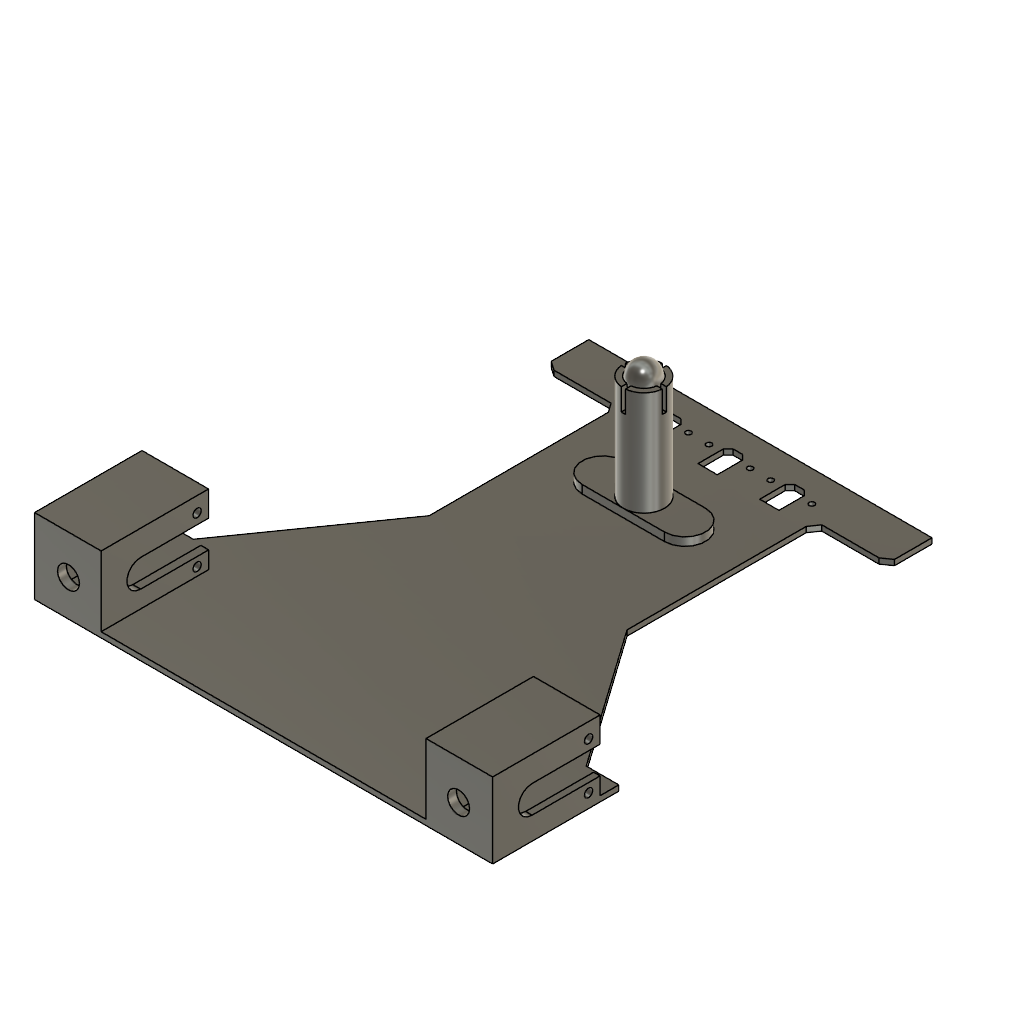
line follower (Autodesk Fusion 360 design; units mm, degrees)
part number: 2026-04-11-10-52-49-664
Autodesk Fusion 360 part; units mm, degrees
note: some values were not read from the file. Set by a fixed rule: which sketch regions a step uses.
sketch "Sketch1" plane through (0, 0, 0) normal (0, 0, 1) x (1, 0, 0)
  line L0 (0, 0) -> (83.525, 0)
  line L1 (83.525, 0) -> (83.525, 46.04)
  line L2 (83.525, 46.04) -> (71.635, 46.04)
  line L3 (71.635, 46.04) -> (36.0768, 96.4755)
  line L4 (36.0768, 96.4755) -> (36.0768, 161.7955)
  line L5 (36.0768, 161.7955) -> (38.4036, 165.1348)
  line L6 (38.4036, 165.1348) -> (59.2636, 165.1348)
  line L7 (59.2636, 165.1348) -> (62.59, 167.48)
  line L8 (62.59, 167.48) -> (62.59, 181.19)
  line L9 (62.59, 181.19) -> (0, 181.19)
  line L10 (0, 181.19) -> (0, 0)
  dimension "d3" = 62.59
  dimension "d4" = 181.19
  dimension "d5" = 13.71
  dimension "d8" = 65.32
  dimension "d9" = 46.04
  dimension "d10" = 83.525
  dimension "d11" = 11.89
  dimension "d12" = 61.71
  dimension "d15" = 4.07
  dimension "d16" = 20.86
  dimension "d18" = 4.07
  constraint coincident L0.start L10.end
  constraint horizontal L0
  constraint perpendicular L0 L1
  constraint perpendicular L1 L2
  constraint perpendicular L0 L4
  constraint perpendicular L4 L6
  constraint perpendicular L3 L7
  constraint perpendicular L0 L8
  constraint perpendicular L8 L9
  constraint perpendicular L0 L10
  measures "d3" distance of L8.end L9.end
  measures "d4" distance of L9.end L0.start
  measures "d5" distance of L7.end L8.end
  measures "d8" distance of L3.end L4.end
  measures "d9" distance of L0.end L1.end
  measures "d10" distance of L0.start L0.end
  measures "d11" distance of L1.end L2.end
  measures "d12" distance of L2.end L3.end
  measures "d15" distance of L6.end L7.end
  measures "d16" distance of L5.end L6.end
  measures "d18" distance of L4.end L5.end
extrude "Extrude1" add sketch "Sketch1" along normal blind 2 makes body 1
mirror "Mirror1" about plane through (0, 0, 0) normal (1, 0, 0) of bodies 1 merged
sketch "Sketch3" plane through (83.525, 0, 0) normal (1, 0, 0) x (0, 1, 0)
  line L0 (0, 0) -> (46.04, 0)
  line L1 (46.04, 0) -> (46.04, 2)
  line L2 (46.04, 2) -> (0, 2)
  line L3 (0, 2) -> (0, 0)
  line L4 (46.04, 2) -> (96.4755, 2)
  line L5 (19.51, 20.5) -> (19.51, 42)
  line L6 (26.51, 20.5) -> (26.51, 42)
  line L7 (19.51, 42) -> (26.51, 42)
  arc A0 (19.51, 20.5) -> (26.51, 20.5) centre (23.01, 20.5) ccw
  dimension "d28" = 7
  dimension "d29" = 18.5
  constraint tangent L5 A0
  constraint tangent L6 A0
  measures "d28" diameter of A0
  measures "d29" distance of A0.centre L4
extrude "Extrude3" cut sketch "Sketch3" against normal blind 2 contours L5 L6 L7 A0 bodies 1
mirror "Mirror2" [no effect]
sketch "Sketch4" plane through (0, 0, 2) normal (0, 0, 1) x (-1, 0, 0)
  line L0 (83.525, -46.04) -> (83.525, 0)
  line L1 (83.525, 0) -> (-83.525, 0)
  line L2 (-83.525, 0) -> (-83.525, -46.04)
  line L3 (-83.525, -46.04) -> (-71.635, -46.04)
  line L4 (-71.635, -46.04) -> (-36.0768, -96.4755)
  line L5 (-36.0768, -96.4755) -> (-36.0768, -161.7955)
  line L6 (-36.0768, -161.7955) -> (-38.4036, -165.1348)
  line L7 (-38.4036, -165.1348) -> (-59.2636, -165.1348)
  line L8 (-59.2636, -165.1348) -> (-62.59, -167.48)
  line L9 (-62.59, -167.48) -> (-62.59, -181.19)
  line L10 (-62.59, -181.19) -> (62.59, -181.19)
  line L11 (62.59, -181.19) -> (62.59, -167.48)
  line L12 (62.59, -167.48) -> (59.2636, -165.1348)
  line L13 (59.2636, -165.1348) -> (38.4036, -165.1348)
  line L14 (38.4036, -165.1348) -> (36.0768, -161.7955)
  line L15 (36.0768, -161.7955) -> (36.0768, -96.4755)
  line L16 (36.0768, -96.4755) -> (71.635, -46.04)
  line L17 (71.635, -46.04) -> (83.525, -46.04)
  line L18 (-3.5, -161.94) -> (3.5, -161.94)
  line L19 (3.5, -161.94) -> (3.5, -172.94)
  line L20 (3.5, -172.94) -> (-3.5, -172.94)
  line L21 (-3.5, -172.94) -> (-3.5, -161.94)
  line L22 (-3.5, -161.94) -> (3.5, -172.94) construction
  line L23 (3.5, -161.94) -> (-3.5, -172.94) construction
  line L24 (-3.5, -171.19) -> (-1.75, -172.94)
  circle A0 centre (-7.5, -169.94) radius 1
  line L25 (0, -167.44) -> (0, -181.19) construction
  circle A1 centre (7.5, -169.94) radius 1
  line L26 (3.5, -171.19) -> (1.75, -172.94)
  circle A2 centre (-30, -169.94) radius 1
  circle A3 centre (-15, -169.94) radius 1
  line L27 (-19, -161.94) -> (-19, -172.94)
  line L28 (-19, -172.94) -> (-26, -172.94)
  line L29 (-26, -172.94) -> (-26, -161.94)
  line L30 (-26, -171.19) -> (-24.25, -172.94)
  line L31 (-26, -161.94) -> (-19, -172.94) construction
  line L32 (-19, -171.19) -> (-20.75, -172.94)
  line L33 (-26, -161.94) -> (-19, -161.94)
  line L34 (-19, -161.94) -> (-26, -172.94) construction
  circle A4 centre (15, -169.94) radius 1
  circle A5 centre (30, -169.94) radius 1
  line L35 (26, -161.94) -> (26, -172.94)
  line L36 (26, -172.94) -> (19, -172.94)
  line L37 (19, -172.94) -> (19, -161.94)
  line L38 (19, -171.19) -> (20.75, -172.94)
  line L39 (19, -161.94) -> (26, -172.94) construction
  line L40 (26, -171.19) -> (24.25, -172.94)
  line L41 (19, -161.94) -> (26, -161.94)
  line L42 (26, -161.94) -> (19, -172.94) construction
  point P0 (0, -167.44)
  point P1 (-22.5, -167.44)
  point P2 (-22.5, -167.44)
  point P3 (22.5, -167.44)
  point P4 (22.5, -167.44)
  dimension "d34" = 7
  dimension "d35" = 11
  dimension "d36" = 8.25
  dimension "d37" = 1.75
  dimension "d38" = 1.75
  dimension "d39" = 2
  dimension "d40" = 11.25
  dimension "d41" = 4
  dimension "d44" = 22.5
  dimension "d45" = 0
  constraint horizontal L18
  constraint perpendicular L18 L19
  constraint parallel L18 L20
  constraint parallel L19 L21
  constraint coincident L22 P0
  constraint coincident L23 P0
  constraint coincident L21 L24.start
  constraint coincident L20 L24.end
  constraint coincident P0 L25.start
  constraint midpoint L10 L25.end
  constraint perpendicular L10 L25
  constraint symmetric L24.start L25 L26.start
  constraint symmetric L24.end L25 L26.end
  constraint symmetric A0 L25 A1
  measures "d34" distance of L18.start L18.end
  measures "d35" distance of L18.end L19.end
  measures "d36" distance of L10 L20
  measures "d37" distance of L20.end L24.end
  measures "d38" distance of L20.end L24.start
  measures "d39" diameter of A0
  measures "d40" distance of L10 A0.centre
  measures "d41" distance of L21 A0.centre
extrude "Extrude4" cut sketch "Sketch4" against normal blind 2 contours L18 L19 L20 L21 L24 L26 | A0 | A1 | A2 | A3 | L27 L28 L29 L30 L32 L33 | A4 | A5 | L35 L36 L37 L38 L40 L41 bodies 1
sketch "Sketch5" plane through (83.525, 0, 0) normal (1, 0, 0) x (0, 1, 0)
  line L0 (0, 0) -> (46.04, 0)
  line L1 (46.04, 0) -> (46.04, 2)
  line L2 (46.04, 2) -> (0, 2)
  line L3 (0, 2) -> (0, 0)
  line L4 (0, 2) -> (24.3, 2)
  line L5 (24.3, 2) -> (24.3, 27.5)
  line L6 (24.3, 27.5) -> (0, 27.5)
  line L7 (0, 27.5) -> (0, 2)
  circle A0 centre (11.9, 13.25) radius 4
  dimension "d48" = 24.3
  dimension "d49" = 25.5
  dimension "d50" = 8
  dimension "d51" = 14.25
  dimension "d53" = 11.9
  constraint horizontal L4
  constraint vertical L5
  constraint horizontal L6
  constraint vertical L7
  constraint coincident L2.end L3.start
  measures "d48" distance of L5.end L6.end
  measures "d49" distance of L2.end L6.end
  measures "d50" diameter of A0
  measures "d51" distance of L6 A0.centre
  measures "d53" distance of L7 A0.centre
extrude "Extrude5" add sketch "Sketch5" against normal blind 39.2 separate body contours L2 L4 L5 L6 L7 makes body 2
sketch "Sketch6" plane through (0, 0, 0) normal (0, -1, 0) x (1, 0, 0)
  line L0 (83.525, 2) -> (83.525, 27.5)
  line L1 (83.525, 27.5) -> (44.325, 27.5)
  line L2 (44.325, 27.5) -> (44.325, 2)
  line L3 (44.325, 2) -> (83.525, 2)
  line L4 (44.325, 8.25) -> (69.125, 8.25)
  arc A0 (69.125, 8.25) -> (69.125, 18.25) centre (69.125, 13.25) ccw
  line L5 (69.125, 18.25) -> (44.325, 18.25)
  arc A1 (44.325, 18.25) -> (44.325, 8.25) centre (44.325, 13.25) ccw
  line L6 (44.325, 13.25) -> (69.125, 13.25) construction
  circle A2 centre (48.525, 22) radius 1.5
  circle A3 centre (48.525, 5) radius 1.5
  dimension "d56" = 6.25
  dimension "d57" = 5
  dimension "d58" = 24.8
  dimension "d59" = 3
  dimension "d60" = 3
  dimension "d61" = 4.2
  dimension "d62" = 4.2
  dimension "d63" = 3
  dimension "d64" = 3.75
  constraint tangent L4 A0
  constraint tangent A0 L5
  constraint parallel L4 L5
  constraint tangent L5 A1
  constraint tangent L4 A1
  constraint perpendicular L2 L6
  constraint coincident L2 A1.centre
  measures "d56" distance of L3 L4
  measures "d57" radius of A0
  measures "d58" distance of A1.centre A0.centre
  measures "d59" diameter of A2
  measures "d60" diameter of A3
  measures "d61" distance of L2 A3.centre
  measures "d62" distance of L2 A2.centre
  measures "d63" distance of L3 A3.centre
  measures "d64" distance of L5 A2.centre
extrude "Extrude6" cut sketch "Sketch6" against normal blind 25 contours L2 L4 A0 L5 | A2 | A3 bodies 2
move_body "Move1" bodies 2 to x (0, -1, 0) y (1, 0, 0) z (0, 0, 1) at (83.525, 83.525, 0)
move_body "Move2" bodies 2 to x (1, 0, 0) y (0, 1, 0) z (0, 0, 1) at (-25, 0, 0)
move_body "Move3" bodies 2 to x (1, 0, 0) y (0, 1, 0) z (0, 0, 1) at (0.7, 0, 0)
sketch "Sketch7" plane through (0, 39.2, 0) normal (0, 1, 0) x (-1, 0, 0)
  line L0 (-59.225, 8.25) -> (-83.525, 8.25)
  line L1 (-83.525, 8.25) -> (-83.525, 2)
  line L2 (-83.525, 2) -> (-59.225, 2)
  line L3 (-59.225, 2) -> (-59.225, 8.25)
  line L4 (-81.175, 2) -> (-62.075, 2)
  line L5 (-62.075, 2) -> (-62.075, 24.65)
  line L6 (-62.075, 24.65) -> (-81.175, 24.65)
  line L7 (-81.175, 24.65) -> (-81.175, 2)
  dimension "d71" = 2.85
  dimension "d72" = 2.35
  dimension "d73" = 22.65
  constraint horizontal L4
  constraint vertical L5
  constraint horizontal L6
  constraint vertical L7
  constraint coincident L2 L4.start
  measures "d71" distance of L3 L5
  measures "d72" distance of L1 L7
  measures "d73" distance of L4 L6
extrude "Extrude7" cut sketch "Sketch7" against normal blind 36 contours L0 L2 L4 L5 L7 | L0 L5 L6 L7 bodies 2
mirror "Mirror3" about plane through (0, 0, 0) normal (1, 0, 0) of bodies 2 makes body 3
sketch "Sketch8" plane through (0, 0, 2) normal (0, 0, 1) x (-1, 0, 0)
  circle A0 centre (15, -169.94) radius 1
  line L0 (1.75, -172.94) -> (-1.75, -172.94)
  line L1 (-1.75, -172.94) -> (-3.5, -171.19)
  line L2 (-3.5, -171.19) -> (-3.5, -161.94)
  line L3 (-3.5, -161.94) -> (3.5, -161.94)
  line L4 (3.5, -161.94) -> (3.5, -171.19)
  line L5 (3.5, -171.19) -> (1.75, -172.94)
  circle A1 centre (-30, -169.94) radius 1
  circle A2 centre (7.5, -169.94) radius 1
  line L6 (24.25, -172.94) -> (20.75, -172.94)
  line L7 (20.75, -172.94) -> (19, -171.19)
  line L8 (19, -171.19) -> (19, -161.94)
  line L9 (19, -161.94) -> (26, -161.94)
  line L10 (26, -161.94) -> (26, -171.19)
  line L11 (26, -171.19) -> (24.25, -172.94)
  circle A3 centre (-15, -169.94) radius 1
  line L12 (-20.75, -172.94) -> (-24.25, -172.94)
  line L13 (-24.25, -172.94) -> (-26, -171.19)
  line L14 (-26, -171.19) -> (-26, -161.94)
  line L15 (-26, -161.94) -> (-19, -161.94)
  line L16 (-19, -161.94) -> (-19, -171.19)
  line L17 (-19, -171.19) -> (-20.75, -172.94)
  circle A4 centre (-7.5, -169.94) radius 1
  circle A5 centre (30, -169.94) radius 1
  line L18 (83.525, 0) -> (-83.525, 0)
  line L19 (-83.525, 0) -> (-83.525, -46.04)
  line L20 (-83.525, -46.04) -> (-71.635, -46.04)
  line L21 (-71.635, -46.04) -> (-36.0768, -96.4755)
  line L22 (-36.0768, -96.4755) -> (-36.0768, -161.7955)
  line L23 (-36.0768, -161.7955) -> (-38.4036, -165.1348)
  line L24 (-38.4036, -165.1348) -> (-59.2636, -165.1348)
  line L25 (-59.2636, -165.1348) -> (-62.59, -167.48)
  line L26 (-62.59, -167.48) -> (-62.59, -181.19)
  line L27 (-62.59, -181.19) -> (62.59, -181.19)
  line L28 (62.59, -181.19) -> (62.59, -167.48)
  line L29 (62.59, -167.48) -> (59.2636, -165.1348)
  line L30 (59.2636, -165.1348) -> (38.4036, -165.1348)
  line L31 (38.4036, -165.1348) -> (36.0768, -161.7955)
  line L32 (36.0768, -161.7955) -> (36.0768, -96.4755)
  line L33 (36.0768, -96.4755) -> (71.635, -46.04)
  line L34 (71.635, -46.04) -> (83.525, -46.04)
  line L35 (83.525, -46.04) -> (83.525, 0)
  line L36 (15, -131.19) -> (-15, -131.19)
  arc A6 (-15, -131.19) -> (-15, -146.19) centre (-15, -138.69) ccw
  line L37 (-15, -146.19) -> (15, -146.19)
  arc A7 (15, -146.19) -> (15, -131.19) centre (15, -138.69) ccw
  line L38 (15, -138.69) -> (-15, -138.69) construction
  point P0 (0, -138.69)
  dimension "d78" = 15
  dimension "d79" = 35
  constraint tangent L36 A6
  constraint tangent A6 L37
  constraint parallel L36 L37
  constraint tangent L37 A7
  constraint tangent L36 A7
  constraint perpendicular L22 L38
  constraint midpoint L38 P0
  measures "d78" diameter of A6
  measures "d79" distance of L27 L37
extrude "Extrude8" add sketch "Sketch8" along normal blind 3 contours L36 A6 L37 A7 bodies 1
sketch "Sketch9" plane through (0, 0, 5) normal (0, 0, 1) x (-1, 0, 0)
  arc A0 (15, -146.19) -> (15, -131.19) centre (15, -138.69) ccw
  line L0 (15, -131.19) -> (-15, -131.19)
  arc A1 (-15, -131.19) -> (-15, -146.19) centre (-15, -138.69) ccw
  line L1 (-15, -146.19) -> (15, -146.19)
  circle A2 centre (0, -138.69) radius 7.5
  dimension "d82" = 15
  dimension "d83" = 7.5
  measures "d82" diameter of A2
  measures "d83" distance of L1 A2.centre
extrude "Extrude9" add sketch "Sketch9" along normal blind 38 separate body contours A2 makes body 4
sphere "SpherePrimitive1" cut diameter 11 placed x (-1, 0, 0) y (0, -1, 0) z (0, 0, 1) at (0, 138.69, 43) bodies 4
sketch "Sketch11" plane through (0, 0, 43) normal (0, 0, 1) x (-1, 0, 0)
  circle A0 centre (0, -138.69) radius 5.5
  circle A1 centre (0, -138.69) radius 7.5
  line L0 (-0.75, -146.19) -> (0.75, -146.19)
  line L1 (0.75, -146.19) -> (0.75, -131.19)
  line L2 (0.75, -131.19) -> (-0.75, -131.19)
  line L3 (-0.75, -131.19) -> (-0.75, -146.19)
  line L4 (-0.75, -146.19) -> (0.75, -131.19) construction
  line L5 (0.75, -146.19) -> (-0.75, -131.19) construction
  line L6 (-7.5, -137.94) -> (7.5, -137.94)
  line L7 (7.5, -137.94) -> (7.5, -139.44)
  line L8 (7.5, -139.44) -> (-7.5, -139.44)
  line L9 (-7.5, -139.44) -> (-7.5, -137.94)
  line L10 (-7.5, -137.94) -> (7.5, -139.44) construction
  line L11 (7.5, -137.94) -> (-7.5, -139.44) construction
  point P0 (0, -138.69)
  point P1 (0, -138.69)
  dimension "d87" = 15
  dimension "d88" = 15
  dimension "d89" = 1.5
  dimension "d90" = 1.5
  constraint horizontal L0
  constraint perpendicular L0 L1
  constraint parallel L0 L2
  constraint parallel L1 L3
  constraint coincident L4 P1
  constraint coincident L5 P1
  constraint coincident P0 A0.centre
  constraint horizontal L6
  constraint perpendicular L6 L7
  constraint parallel L6 L8
  constraint parallel L7 L9
  constraint coincident L10 P1
  constraint coincident L11 P1
  constraint coincident P1 P0
  measures "d87" distance of L0.end L1.end
  measures "d88" distance of L6.start L6.end
  measures "d89" distance of L0.start L0.end
  measures "d90" distance of L6.start L8.end
extrude "Extrude10" cut sketch "Sketch11" against normal blind 8 contours A0 L1 L6 L8 | A0 A1 L6 L8 | A0 L1 L3 L6 | A0 A1 L1 L3 | L1 L3 L6 L8 | A0 A1 L1 L3 | A0 L1 L3 L8 | A0 L3 L6 L8 | A0 A1 L6 L8 bodies 4
sphere "SpherePrimitive2" add diameter 10.5 placed x (-1, 0, 0) y (0, -1, 0) z (0, 0, 1) at (0, 138.69, 43) separate body makes body 5
combine "Combine1" operation add target body 1 tool bodies 2 3
